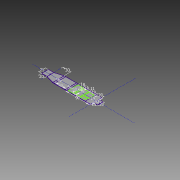
# Autodesk Inventor part: BandSide
Saved by Autodesk Inventor 2016 (Build 200138000, 138)
## iProperties
Created: 2015-04-10
Part Number: BandSide
Material: Generic
Document SubType Name: Modeling
Designer: Erin
Density: 1 g/cm^3
Appearance: Default
Author: Erin
Autodesk Inventor part; units mm, degrees
ref_plane "YZ Plane" through (0, 0, 0) normal (1, 0, 0) x (0, 1, 0)
ref_plane "XZ Plane" through (0, 0, 0) normal (0, 1, 0) x (-1, 0, 0)
ref_plane "XY Plane" through (0, 0, 0) normal (0, 0, 1) x (1, 0, 0)
sketch "Sketch1" plane through (0, 0, 0) normal (0, 0, 1) x (1, 0, 0)
  line L0 (-90, 21.5) -> (0, 21.5)
  line L1 (0, 21.5) -> (0, -21.5)
  line L2 (0, -21.5) -> (-90, -21.5)
  line L3 (-90, -21.5) -> (-90, 21.5)
  line L4 (-90, 21.5) -> (-142, 21.5)
  line L5 (-142, 21.5) -> (-142, -21.5)
  line L6 (-142, -21.5) -> (-90, -21.5)
  line L7 (-90, -21.5) -> (-90, 21.5)
  line L8 (-96, 21.5) -> (-96, -21.5)
  line L9 (-136, 21.5) -> (-136, -21.5)
  line L10 (-172, 39.3338) -> (-172, -34.4361) construction
  line L11 (-172, 12.5) -> (-192, 12.5)
  line L12 (-192, 12.5) -> (-192, -12.5)
  line L13 (-192, -12.5) -> (-172, -12.5)
  line L14 (-172, -12.5) -> (-172, 12.5)
  line L15 (-237.0195, 0) -> (143.1564, 0) construction
  line L16 (0, 148.4042) -> (0, -100.7046) construction
  line L17 (-172, 12.5) -> (-142, 21.5)
  line L18 (-172, -12.5) -> (-142, -21.5)
  line L19 (-20, 21.5) -> (-20, -21.5)
  line L20 (0, 10) -> (15, 10)
  line L21 (15, 10) -> (15, -10)
  line L22 (15, -10) -> (0, -10)
  line L23 (0, -10) -> (0, 10)
  line L24 (-63.7943, -15.2321) -> (-63.7943, 15.4179)
  line L25 (-63.7943, 15.4179) -> (-44.6843, 15.4179)
  line L26 (-44.6843, 15.4179) -> (-44.6843, -15.2321)
  line L27 (-44.6843, -15.2321) -> (-63.7943, -15.2321)
  line L28 (-86.4422, 19.0102) -> (-68.4422, 19.0102)
  line L29 (-68.4422, 19.0102) -> (-68.4422, -18.9898)
  line L30 (-68.4422, -18.9898) -> (-86.4422, -18.9898)
  line L31 (-86.4422, -18.9898) -> (-86.4422, 19.0102)
  line L32 (-41.3198, 14.7798) -> (-22.3198, 14.7798)
  line L33 (-22.3198, 14.7798) -> (-22.3198, -4.2202)
  line L34 (-22.3198, -4.2202) -> (-41.3198, -4.2202)
  line L35 (-41.3198, -4.2202) -> (-41.3198, 14.7798)
  line L36 (-41.3198, -7.7055) -> (-24.4109, -7.7055)
  line L37 (-24.4109, -7.7055) -> (-24.4109, -17)
  line L38 (-24.4109, -17) -> (-41.3198, -17)
  line L39 (-41.3198, -17) -> (-41.3198, -7.7055)
  point P0 (0, 0)
  point P1 (0, 0)
  point P2 (-172, 0)
  point P3 (15, 0)
  dimension "d0" = 90
  dimension "d1" = 43
  dimension "d2" = 6
  dimension "d3" = 6
  dimension "d5" = 40
  dimension "d6" = 30
  dimension "d7" = 20
  dimension "d8" = 25
  dimension "d23" = 20
  dimension "d34" = 15
  dimension "d35" = 20
  dimension "d36" = 19
  dimension "d37" = 19
  dimension "d38" = 30.65
  dimension "d39" = 19.11
  dimension "d40" = 38
  dimension "d41" = 18
  constraints: 80 end point, 17 parallel, 13 perpendicular, 8 horizontal, 8 point on line, 3 midpoint, 2 collinear, 2 horizontal alignment, 1 coincident, 1 vertical
  measures "d0" distance of L1.end L2.end
  measures "d1" distance of L0.end L1.end
  measures "d2" distance between parallel lines of L7 L8
  measures "d3" distance between parallel lines of L5 L9
  measures "d5" distance between parallel lines of L8 L9
  measures "d6" distance between parallel lines of L10 L5
  measures "d7" distance of L13.end L12.end
  measures "d8" distance of L12.end L11.end
  measures "d23" distance between parallel lines of L19 L1
  measures "d34" distance of L21.end L22.end
  measures "d35" distance of L20.end L21.end
  measures "d36" distance of L32.start L32.end
  measures "d37" distance of L32.end L33.end
  measures "d38" distance of L24.start L24.end
  measures "d39" distance of L24.end L25.end
  measures "d40" distance of L28.end L29.end
  measures "d41" distance of L28.start L28.end
extrude "Extrusion1" add sketch "Sketch1" along normal blind 0.2 contours L0 L19 L2 L3 | L3 L6 L8 L4 | L0 L1 L2 L19 | L8 L6 L9 L4 | L9 L6 L5 L4 | L20 L21 L22 L1 | L5 L18 L14 L17 | L14 L13 L12 L11 | L24 L25 L26 L27 | L28 L29 L30 L31 | L32 L33 L34 L35 | L36 L37 L38 L39
extrude "Extrusion3" add sketch "Sketch1" along normal blind 0.4 contours L0 L1 L2 L19 | L20 L21 L22 L1
extrude "Extrusion4" add sketch "Sketch1" along normal blind 0.4 contours L14 L13 L12 L11
equation "\"d19\" = material"
equation "\"d30\" = 2 * material"
equation "\"d32\" = 2 * material"
equation "\"material\" = 0.2"
body "Solid1"
